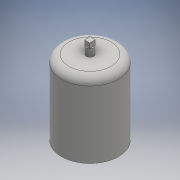
# Autodesk Inventor part: Lifting Pad Motor Redo
Saved by Autodesk Inventor 2016 (Build 200138000, 138)
## iProperties
Created: 2016-02-23
Part Number: Lifting Pad Motor Redo
Material: Generic
Document SubType Name: Modeling
Designer: Kenneth Daniel
Density: 1 g/cm^3
Appearance: Default
Author: Kenneth Daniel
Autodesk Inventor part; units mm, degrees
ref_plane "YZ Plane" through (0, 0, 0) normal (1, 0, 0) x (0, 1, 0)
ref_plane "XZ Plane" through (0, 0, 0) normal (0, 1, 0) x (-1, 0, 0)
ref_plane "XY Plane" through (0, 0, 0) normal (0, 0, 1) x (1, 0, 0)
sketch "Sketch1" plane through (0, 0, 0) normal (0, 0, 1) x (1, 0, 0)
  circle A0 centre (0, 0) radius 11.5
  dimension "d0" = 23
  constraints: 1 centre point, 1 coincident
  measures "d0" diameter of A0
extrude "Extrusion1" add sketch "Sketch1" along normal blind 30
fillet "Fillet1" radius 3 1 edges at (-11.5, 0, 30)
sketch "Sketch2" plane through (0, 0, 30) normal (0, 0, 1) x (1, 0, 0)
  circle A0 centre (0, 0) radius 1.5
  dimension "d4" = 3
  constraints: 1 centre point, 1 coincident
  measures "d4" diameter of A0
extrude "Extrusion2" add sketch "Sketch2" along normal blind 5
sketch "Sketch3" plane through (0, 0, 35) normal (0, 0, 1) x (1, 0, 0)
  circle A0 centre (0, 0) radius 1.5 projected
  line L0 (-0.9939, -1.1235) -> (0.9939, -1.1235)
  line L1 (0.9939, -1.1235) -> (0.9939, 1.1235)
  line L2 (0.9939, 1.1235) -> (-0.9939, 1.1235)
  line L3 (-0.9939, 1.1235) -> (-0.9939, -1.1235)
  line L4 (-0.9939, -1.1235) -> (0.9939, 1.1235) construction
  line L5 (0.9939, -1.1235) -> (-0.9939, 1.1235) construction
  constraints: 12 end point, 2 midpoint, 2 parallel, 1 horizontal, 1 perpendicular, 2 other
extrude "Extrusion3" cut sketch "Sketch3" against normal blind 2 contours A0 L1 | L2 A0 | A0 L0 | L3 A0
body "Solid1"
